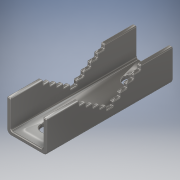
# Autodesk Inventor part: 0070.2 - Abraçadeira suporte
Saved by Autodesk Inventor 2019.4 (Build 234330000, 330)
## iProperties
Created: 2021-04-22
Part Number: 0070.2 - Abraçadeira suporte
Material: Aço, carbono
Document SubType Name: Modeling
Designer: Lattes
Density: 7.85 g/cm^3
Appearance: Semipolido
Author: Lattes
Autodesk Inventor part; units mm, degrees
ref_plane "YZ Plane" through (0, 0, 0) normal (1, 0, 0) x (0, 1, 0)
ref_plane "XZ Plane" through (0, 0, 0) normal (0, 1, 0) x (-1, 0, 0)
ref_plane "XY Plane" through (0, 0, 0) normal (0, 0, 1) x (1, 0, 0)
sketch "Esboço1" plane through (0, 0, 0) normal (0, 0, 1) x (1, 0, 0)
  line L0 (0, 0) -> (10, 0)
  line L1 (10, 0) -> (10, 16)
  line L2 (10, 16) -> (8, 16)
  line L3 (8, 16) -> (8, 2)
  line L4 (8, 2) -> (0, 2)
  line L5 (0, 0) -> (-10, 0)
  line L6 (-10, 0) -> (-10, 16)
  line L7 (-10, 16) -> (-8, 16)
  line L8 (-8, 16) -> (-8, 2)
  line L9 (-8, 2) -> (0, 2)
  dimension "d4" = 10
  dimension "d5" = 16
  dimension "d6" = 2
  dimension "d7" = 14
  dimension "d8" = 8
  constraints: 20 end point, 3 horizontal, 2 perpendicular
  measures "d4" distance of L0.start L0.end
  measures "d5" distance of L0.end L1.end
  measures "d6" distance of L1.end L2.end
  measures "d7" distance of L2.end L3.end
  measures "d8" distance of L3.end L4.end
extrude "Extrusão1" add sketch "Esboço1" along normal blind 63
sketch "Esboço2" plane through (-10, 0, 0) normal (0, -1, 0) x (1, 0, 0)
  line L0 (10, 0) -> (10, 63)
  line L1 (10, 31.5) -> (10, 11)
  line L2 (10, 11) -> (10, 52)
  circle A0 centre (10, 52) radius 3.5
  circle A1 centre (10, 11) radius 3.5
  dimension "d11" = 20.5
  dimension "d12" = 41
  dimension "d13" = 7
  dimension "d14" = 7
  constraints: 6 end point, 2 centre point, 2 coincident, 2 point on line, 1 midpoint, 1 vertical
  measures "d11" distance of L1.start L1.end
  measures "d12" distance of L1.end L2.end
  measures "d13" diameter of A0
  measures "d14" diameter of A1
extrude "Extrusão2" cut sketch "Esboço2" against normal blind 63
sketch "Esboço3" plane through (10, 0, 0) normal (1, 0, 0) x (0, 0, -1)
  line L0 (0, 0) -> (-63, 0) projected
  line L1 (-14.5, 0) -> (-14.5, 2) projected
  line L2 (0, 2) -> (-63, 2) projected
  line L3 (-31.5, 5) -> (-29.8, 5)
  line L4 (-29.8, 5) -> (-29.8, 7.2)
  line L5 (-29.8, 7.2) -> (-26.4, 7.2)
  line L6 (-26.4, 7.2) -> (-26.4, 9.4)
  line L7 (-26.4, 9.4) -> (-23, 9.4)
  line L8 (-23, 9.4) -> (-23, 11.6)
  line L9 (-23, 11.6) -> (-19.6, 11.6)
  line L10 (-19.6, 11.6) -> (-19.6, 13.8)
  line L11 (-19.6, 13.8) -> (-16.2, 13.8)
  line L12 (-16.2, 13.8) -> (-16.2, 16)
  line L13 (-31.5, 5) -> (-33.2, 5)
  line L14 (-33.2, 5) -> (-33.2, 7.2)
  line L15 (-33.2, 7.2) -> (-36.6, 7.2)
  line L16 (-36.6, 7.2) -> (-36.6, 9.4)
  line L17 (-36.6, 9.4) -> (-40, 9.4)
  line L18 (-40, 9.4) -> (-40, 11.6)
  line L19 (-40, 11.6) -> (-43.4, 11.6)
  line L20 (-43.4, 11.6) -> (-43.4, 13.8)
  line L21 (-43.4, 13.8) -> (-46.8, 13.8)
  line L22 (-46.8, 13.8) -> (-46.8, 16)
  line L23 (-46.8, 16) -> (-16.2, 16)
  dimension "d18" = 1.7
  dimension "d19" = 2.2
  dimension "d20" = 3.4
  dimension "d21" = 2.2
  dimension "d22" = 3.4
  dimension "d23" = 2.2
  dimension "d24" = 3.4
  dimension "d25" = 2.2
  dimension "d26" = 3.4
  constraints: 42 end point, 8 perpendicular, 2 horizontal
  measures "d18" distance of L3.start L3.end
  measures "d19" distance of L3.end L4.end
  measures "d20" distance of L4.end L5.end
  measures "d21" distance of L5.end L6.end
  measures "d22" distance of L6.end L7.end
  measures "d23" distance of L7.end L8.end
  measures "d24" distance of L8.end L9.end
  measures "d25" distance of L9.end L10.end
  measures "d26" distance of L10.end L11.end
extrude "Extrusão3" cut sketch "Esboço3" against normal blind 63
fillet "Arredondamento1" radius 2 2 edges at (-10, 0, 31.5) (10, 0, 31.5)
fillet "Arredondamento2" radius 1 2 edges at (-8, 2, 31.5) (8, 2, 31.5)
fillet "Arredondamento3" radius 0.5 36 edges at (-3.5, 2, 52) (-3.5, 0, 52) (-3.5, 0, 11) (-3.5, 2, 11) (0, 2, 63) (7.7071, 2.2929, 63) (8, 9.5, 63) (-8, 9.5, 63) (-7.7071, 2.2929, 63) (-9.4142, 0.5858, 63) (0, 0, 63) (9.4142, 0.5858, 63) (10, 9, 63) (-10, 9, 63) (9.4142, 0.5858, 0) (10, 9, 0) (-9.4142, 0.5858, 0) (-10, 9, 0) (0, 0, 0) (-7.7071, 2.2929, 0) (-8, 9.5, 0) (7.7071, 2.2929, 0) (8, 9.5, 0) (0, 2, 0) (-8, 16, 54.9) (-10, 16, 54.9) (-9, 16, 63) (8, 16, 54.9) (10, 16, 54.9) (9, 16, 63) (10, 16, 8.1) (8, 16, 8.1) (9, 16, 0) (-8, 16, 8.1) (-10, 16, 8.1) (-9, 16, 0)
fillet "Arredondamento4" radius 0.5 63 edges at (9, 13.8, 46.8) (8.1464, 15.8536, 46.8) (8, 14.65, 46.8) (9.8536, 15.8536, 46.8) (10, 14.65, 46.8) (9, 16, 46.8) (10, 13.8, 45.1) (8, 13.8, 45.1) (9, 13.8, 43.4) (9, 11.6, 43.4) (10, 12.7, 43.4) (8, 12.7, 43.4) (8, 11.6, 41.7) (10, 11.6, 41.7) (9, 11.6, 40) (8, 10.5, 40) (10, 10.5, 40) (9, 9.4, 40) (10, 9.4, 38.3) (8, 9.4, 38.3) (9, 9.4, 36.6) (8, 8.3, 36.6) (10, 8.3, 36.6) (9, 7.2, 36.6) (8, 7.2, 34.9) (10, 7.2, 34.9) (9, 7.2, 33.2) (8, 6.1, 33.2) (10, 6.1, 33.2) (9, 5, 33.2) (-9, 5, 29.8) (9, 5, 29.8) (8, 5, 31.5) (10, 5, 31.5) (9.8536, 15.8536, 16.2) (9, 16, 16.2) (8.1464, 15.8536, 16.2) (8, 14.65, 16.2) (10, 14.65, 16.2) (9, 13.8, 16.2) (8, 13.8, 17.9) (10, 13.8, 17.9) (9, 13.8, 19.6) (8, 12.7, 19.6) (10, 12.7, 19.6) (9, 11.6, 19.6) (8, 11.6, 21.3) (10, 11.6, 21.3) (9, 11.6, 23) (8, 10.5, 23) (10, 10.5, 23) (9, 9.4, 23) (8, 9.4, 24.7) (10, 9.4, 24.7) (9, 9.4, 26.4) (8, 8.3, 26.4) (10, 8.3, 26.4) (9, 7.2, 26.4) (8, 7.2, 28.1) (10, 7.2, 28.1) (9, 7.2, 29.8) (8, 6.1, 29.8) (10, 6.1, 29.8)
fillet "Arredondamento5" radius 0.5 61 edges at (-8.1464, 15.8536, 16.2) (-8, 14.65, 16.2) (-9.8536, 15.8536, 16.2) (-10, 14.65, 16.2) (-9, 16, 16.2) (-9, 13.8, 16.2) (-8, 13.8, 17.9) (-10, 13.8, 17.9) (-9, 13.8, 19.6) (-8, 12.7, 19.6) (-10, 12.7, 19.6) (-9, 11.6, 19.6) (-8, 11.6, 21.3) (-10, 11.6, 21.3) (-9, 11.6, 23) (-8, 10.5, 23) (-10, 10.5, 23) (-9, 9.4, 23) (-8, 9.4, 24.7) (-10, 9.4, 24.7) (-9, 9.4, 26.4) (-8, 8.3, 26.4) (-10, 8.3, 26.4) (-9, 7.2, 26.4) (-8, 7.2, 28.1) (-10, 7.2, 28.1) (-9, 7.2, 29.8) (-8, 6.35, 29.8) (-10, 6.35, 29.8) (-9, 5, 33.2) (-8, 5, 31.75) (-10, 5, 31.75) (-9, 7.2, 33.2) (-8, 6.1, 33.2) (-10, 6.1, 33.2) (-9.8536, 15.8536, 46.8) (-10, 14.65, 46.8) (-8.1464, 15.8536, 46.8) (-8, 14.65, 46.8) (-9, 16, 46.8) (-9, 13.8, 46.8) (-8, 13.8, 45.1) (-10, 13.8, 45.1) (-9, 13.8, 43.4) (-8, 12.7, 43.4) (-10, 12.7, 43.4) (-9, 11.6, 43.4) (-8, 11.6, 41.7) (-10, 11.6, 41.7) (-9, 11.6, 40) (-8, 10.5, 40) (-10, 10.5, 40) (-9, 9.4, 40) (-8, 9.4, 38.3) (-10, 9.4, 38.3) (-9, 9.4, 36.6) (-9, 7.2, 36.6) (-8, 8.3, 36.6) (-10, 8.3, 36.6) (-10, 7.2, 34.9) (-8, 7.2, 34.9)
